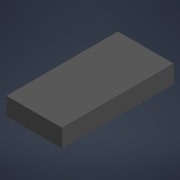
# Autodesk Inventor part: 110033226_ipt_08_平滑面(2x1)
Saved by Autodesk Inventor 2022 (Build 260153000, 153)
## iProperties
Created: 2022-06-22
Part Number: 110033226_ipt_08_平滑面(2x1)
Material: 一般
Document SubType Name: Modeling
Designer: User
Density: 1 g/cm^3
Appearance: 預設
Author: User
Autodesk Inventor part; units mm, degrees
ref_plane "YZ Plane" through (0, 0, 0) normal (1, 0, 0) x (0, 1, 0)
ref_plane "XZ Plane" through (0, 0, 0) normal (0, 1, 0) x (-1, 0, 0)
ref_plane "XY Plane" through (0, 0, 0) normal (0, 0, 1) x (1, 0, 0)
sketch "草圖1" plane through (0, 0, 0) normal (0, 1, 0) x (-1, 0, 0)
  line L0 (2.5, 5) -> (-2.5, 5)
  line L1 (-2.5, 5) -> (-2.5, -5)
  line L2 (-2.5, -5) -> (2.5, -5)
  line L3 (2.5, -5) -> (2.5, 5)
  circle A0 centre (0, 2.5) radius 1.7
  line L4 (2.5, 0) -> (-2.5, 0) construction
  circle A1 centre (0, -2.5) radius 1.7
  point P0 (0, 0)
  point P1 (0, 5)
  dimension "d0" = 5
  dimension "d1" = 10
  dimension "d2" = 3.4
  dimension "d3" = 2.5
  dimension "d4" = 2.5
  constraints: 10 end point, 3 midpoint, 2 centre point, 2 parallel, 1 horizontal, 1 horizontal alignment, 1 perpendicular, 1 symmetric about line, 1 vertical alignment, 1 other
  measures "d0" distance of L2.end L1.end
  measures "d1" distance of L1.end L0.end
  measures "d2" diameter of A0
  measures "d3" distance from line of L3 A0.centre
  measures "d4" distance from line of L0 A0.centre
extrude "擠出1" add sketch "草圖1" along normal blind 1.6 contours L3 L2 L1 L0 | A0 | A1
extrude "擠出2" cut sketch "草圖1" along normal blind 1.5 contours A0 | A1
